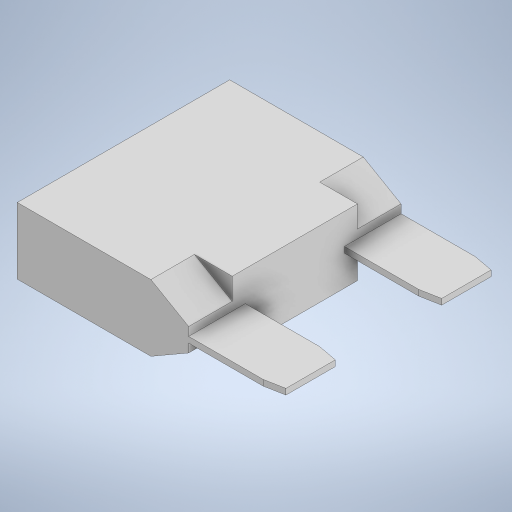
# Autodesk Inventor part: C0-1-01-circuitBreaker
Saved by Autodesk Inventor 2023 (Build 270158000, 158)
## iProperties
Created: 2023-02-23
Part Number: C0-1-01-circuitBreaker
Material: Generic
Document SubType Name: Modeling
Designer: t205b
Density: 1 g/cm^3
Appearance: Default
Author: t205b
Autodesk Inventor part; units mm, degrees
ref_plane "YZ Plane" through (0, 0, 0) normal (1, 0, 0) x (0, 1, 0)
ref_plane "XZ Plane" through (0, 0, 0) normal (0, 1, 0) x (-1, 0, 0)
ref_plane "XY Plane" through (0, 0, 0) normal (0, 0, 1) x (1, 0, 0)
sketch "Sketch1" plane through (0, 0, 0) normal (0, 1, 0) x (-1, 0, 0)
  line L0 (23.6, 14.625) -> (23.6, -14.625)
  line L1 (23.6, -14.625) -> (-10.25, -14.625)
  line L2 (-12.9, -14.125) -> (-12.9, -7.325)
  line L3 (-10.25, -6.825) -> (0, -6.825)
  line L4 (0, -6.825) -> (0, 6.825)
  line L5 (0, 6.825) -> (-10.25, 6.825)
  line L6 (-12.9, 7.325) -> (-12.9, 14.125)
  line L7 (-10.25, 14.625) -> (23.6, 14.625)
  line L8 (30.9, 0) -> (-20.2, 0) projected
  line L9 (-12.9, 14.125) -> (-10.25, 14.625)
  line L10 (-12.9, 7.325) -> (-10.25, 6.825)
  line L11 (-12.9, -7.325) -> (-10.25, -6.825)
  line L12 (-12.9, -14.125) -> (-10.25, -14.625)
  point P0 (-12.9, 6.825)
  point P1 (-12.9, 14.625)
  dimension "d0" = 29.25
  dimension "d1" = 23.6
  dimension "d2" = 7.8
  dimension "d3" = 12.9
  dimension "d14" = 6.825
  dimension "d15" = 13.65
  dimension "d16" = 6.8
  dimension "d17" = 6.8
  dimension "d18" = 2.65
  dimension "d19" = 2.65
  dimension "d20" = 2.65
  dimension "d21" = 2.65
  dimension "d22" = 0.5
  dimension "d23" = 0.5
  constraints: 24 end point, 5 perpendicular, 2 equal length, 2 horizontal alignment, 2 point on line, 2 vertical, 1 parallel, 1 other
  measures "d0" distance between parallel lines of L1 L7
  measures "d1" distance between parallel lines of L0 L4
  measures "d2" distance between parallel lines of L1 L3
  measures "d3" distance between parallel lines of L4 L2
  measures "d14" distance of the line from the sketch origin of L3
  measures "d15" distance of L3.end L4.end
  measures "d16" distance of L6.start L6.end
  measures "d17" distance of L2.start L2.end
  measures "d18" distance from line of L7.start L6
  measures "d19" distance from line of L5.end L6
  measures "d20" distance from line of L1.end L2
  measures "d21" distance from line of L3.start L2
  measures "d22" distance from line of L2.start L1
  measures "d23" distance from line of L6.start L5
extrude "Extrusion1" add sketch "Sketch1" along normal mid plane 0.8
sketch "Sketch2" plane through (0, 0, 0) normal (0, 1, 0) x (-1, 0, 0)
  line L0 (23.6, -14.625) -> (23.6, 14.625) projected
  line L1 (23.6, 14.625) -> (-10.25, 14.625) projected
  line L2 (0, 0) -> (0, -6.825) projected
  line L3 (0, 0) -> (0, 14.625)
  line L4 (0, -6.825) -> (0, -14.625)
  line L5 (-10.25, -14.625) -> (23.6, -14.625) projected
  point P0 (-12.9, 14.625)
  constraints: 4 end point, 2 point on line, 1 perpendicular
extrude "Extrusion2" add sketch "Sketch2" along normal mid plane 9.15
sketch "Sketch3" plane through (0, -0.4, 14.625) normal (0, 0, 1) x (1, 0, 0)
  line L0 (-23.6, 4.975) -> (0, 4.975) projected
  line L1 (0, 0.8) -> (0, 4.975) projected
  line L2 (-5.2, 4.975) -> (0, 1.975)
  point P0 (0, 0.4)
  dimension "d10" = 5.2
  dimension "d11" = 3
  constraints: 2 end point, 2 point on line
  measures "d10" distance from line of L1 L2.start
  measures "d11" distance from line of L0 L2.end
extrude "Extrusion3" cut sketch "Sketch3" against normal blind 6
mirror "Mirror1" about plane through (0, 0, 0) normal (0, 0, 1) of "Extrusion3"
mirror "Mirror2" about plane through (0, 0, 0) normal (0, 1, 0) of "Extrusion3", "Mirror1"
equation "\"d14\" = 0.5 * d15"
body "Solid1"
